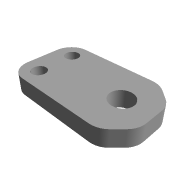
# Autodesk Inventor part: 100025
Saved by Autodesk Inventor 2020.1 (Build 241239000, 239)
## iProperties
Company: AUTODESK, INC.
Part Number: 100025
Document SubType Name: Modeling
Created: 2003-06-12
Designer: SCHNEIDER K.
Material: STEEL - HIGH GRADE ALLOY
Description: HINGE PLATE
Project: ADSK-000-000000
Density: 7.86 g/cm^3
Appearance: Default
Control State: 0
Master: False
Checked Out: False
Shininess: 64.0
Length Units: 11269
Angle Units: 11279
Time Units: 11290
Mass Units: 11283
Length Display Precision: 2
Angle Display Precision: 2
Compacted: True
Density: 0.0
Volumn: 0.0
Area: 0.0
PropertySet Name: Model Information
Title: PLATE
Author: schneik
Revision Number: -
Autodesk Inventor part; units mm, degrees
ref_plane "YZ Plane" through (0, 0, 0) normal (1, 0, 0) x (0, 1, 0)
ref_plane "XZ Plane" through (0, 0, 0) normal (0, 1, 0) x (-1, 0, 0)
ref_plane "XY Plane" through (0, 0, 0) normal (0, 0, 1) x (1, 0, 0)
sketch "スケッチ2" plane through (0, 0, 0) normal (0, 0, 1) x (1, 0, 0)
  line L0 (-50, 19) -> (5, 19)
  line L1 (15, 9) -> (15, -9)
  line L2 (5, -19) -> (-50, -19)
  line L3 (-50, -19) -> (-50, 19)
  line L4 (15, 9) -> (5, 19)
  line L5 (15, -9) -> (5, -19)
  point P0 (15, -19)
  point P1 (15, 19)
  point P2 (0, 0)
  dimension "d2" = 10
  dimension "d3" = 10
  dimension "d4" = 10
  dimension "d5" = 10
  dimension "d6" = 38
  dimension "d7" = 65
  dimension "d34" = 19
  dimension "d36" = 50
  constraints: 12 end point, 4 point on line, 2 parallel, 1 horizontal, 1 perpendicular
  measures "d2" distance of L1.start point (15, 19)
  measures "d3" distance of L0.end point (15, 19)
  measures "d4" distance of L1.end point (15, -19)
  measures "d5" distance of L2.start point (15, -19)
  measures "d6" distance between parallel lines of L2 L0
  measures "d7" distance between parallel lines of L1 L3
  measures "d34" distance from line of L0 point (0, 0)
  measures "d36" distance from line of point (0, 0) L3
extrude "押し出し2" add sketch "スケッチ2" along normal mid plane 9
sketch "スケッチ4" plane through (0, 0, -4.5) normal (0, 0, -1) x (-1, 0, 0)
  line L0 (50, 19) -> (50, -19) projected
  line L1 (50, -19) -> (-5, -19) projected
  point P0 (40, -10)
  point P1 (40, 10)
  dimension "d24" = 10
  dimension "d25" = 9
  dimension "d26" = 20
  constraints: 1 vertical alignment
  measures "d24" distance from line of point (40, -10) L0
  measures "d25" distance from line of point (40, -10) L1
  measures "d26" distance of point (40, 10) point (40, -10)
hole "穴2" at (-40, -10, -4.5) at (-40, 10, -4.5) direction (0, 0, 1) diameter 8 end through all
sketch "スケッチ5" plane through (0, 0, 4.5) normal (0, 0, 1) x (1, 0, 0)
  point P0 (0, 0)
  point P1 (0, 0)
  constraints: 1 coincident
hole "穴3" at (0, 0, 4.5) direction (0, 0, -1) diameter 12 end through all
fillet "Fillet1" radius 10 6 edges at (-50, 19, 0) (-50, -19, 0) (5, -19, 0) (15, -9, 0) (15, 9, 0) (5, 19, 0)
equation "\"d3\" = d2"
equation "\"d4\" = d2"
equation "\"d5\" = d4"
equation "\"d34\" = 0.5 * d6"
body "Solid1"
